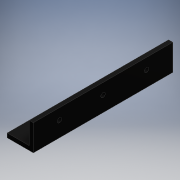
# Autodesk Inventor part: Horn_Bracket
Saved by Autodesk Inventor 2016 (Build 200138000, 138)
## iProperties
Created: 2016-05-21
Part Number: Horn_Bracket
Material: Steel, Cast
Document SubType Name: Modeling
Designer: agmle
Density: 7.85 g/cm^3
Appearance: Glossy - Black
Mass: 1504.55 g
Surface Area: 548.079 cm^2
Volume: 191.662 cm^3
Mounting_Hole_Spacing: 82.800 mm
Mounting_Hole_Diameter: 8.450 mm
Author: agmle
Autodesk Inventor part; units mm, degrees
ref_plane "YZ Plane" through (0, 0, 0) normal (1, 0, 0) x (0, 1, 0)
ref_plane "XZ Plane" through (0, 0, 0) normal (0, 1, 0) x (-1, 0, 0)
ref_plane "XY Plane" through (0, 0, 0) normal (0, 0, 1) x (1, 0, 0)
sketch "Sketch1" plane through (0, 0, 0) normal (0, 1, 0) x (-1, 0, 0)
  line L0 (0, 0) -> (0, 49.7)
  line L1 (0, 49.7) -> (8, 49.7)
  line L2 (8, 49.7) -> (8, 8)
  line L3 (8, 8) -> (49.7, 8)
  line L4 (49.7, 8) -> (49.7, 0)
  line L5 (49.7, 0) -> (0, 0)
  dimension "d0" = 49.7
  dimension "d1" = 8
  constraints: 12 end point, 6 perpendicular, 1 parallel, 1 vertical
  measures "d0" distance between parallel lines of L0 L4
  measures "d1" distance between parallel lines of L0 L2
extrude "Extrusion1" add sketch "Sketch1" along normal blind 265
sketch "Sketch2" plane through (0, 0, 0) normal (0, 0, -1) x (-1, 0, 0)
  line L0 (49.7, 0) -> (0, 0) construction
  line L1 (49.7, 0) -> (49.7, 265) construction
  line L2 (0, 265) -> (49.7, 265) construction
  line L3 (0, 0) -> (0, 265) construction
  line L4 (31, 0) -> (31, 265) construction
  line L5 (0, 265) -> (49.7, 265) construction
  point P0 (31, 231)
  point P1 (31, 205)
  point P2 (31, 60)
  point P3 (31, 34)
  dimension "d4" = 26
  dimension "d5" = 26
  dimension "d6" = 34
  dimension "d7" = 34
  dimension "d8" = 31
  constraints: 6 point on line, 2 end point, 1 perpendicular
  measures "d4" distance of point (31, 34) point (31, 60)
  measures "d5" distance of point (31, 231) point (31, 205)
  measures "d6" distance from line of L2 point (31, 231)
  measures "d7" distance from line of L0 point (31, 34)
  measures "d8" distance between parallel lines of L3 L4
hole "Hole1" at (-31, 231, 0) at (-31, 205, 0) at (-31, 60, 0) at (-31, 34, 0) direction (0, 0, 1) diameter 5.5 depth 8 tip angle 118 clearance for "Hex Head Bolt" size "M5" standard "Ansi Metric M Profile"
sketch "Sketch3" plane through (0, 0, 49.7) normal (1, 0, 0) x (0, 0, -1)
  line L0 (49.7, 0) -> (0, 0) construction
  line L1 (49.7, 0) -> (49.7, 265) construction
  line L2 (0, 265) -> (49.7, 265) construction
  line L3 (0, 0) -> (0, 265) construction
  line L4 (0, 0) -> (41.7, 0) construction
  line L5 (20.8, 0) -> (20.8, 265) construction
  point P0 (20.8, 132.5)
  point P1 (20.8, 215.3)
  point P2 (20.8, 49.7)
  dimension "d16" = 20.8
  dimension "Mounting_Hole_Spacing" = 82.8
  dimension "d18" = 82.8
  constraints: 4 point on line, 2 end point, 1 midpoint, 1 perpendicular
  measures "d16" distance between parallel lines of L3 L5
  measures "Mounting_Hole_Spacing" distance of point (20.8, 132.5) point (20.8, 49.7)
  measures "d18" distance of point (20.8, 215.3) point (20.8, 132.5)
hole "Hole2" at (0, 132.5, 28.9) at (0, 215.3, 28.9) at (0, 49.7, 28.9) direction (-1, 0, 0) diameter 8.45 end through all
equation "\"d4\" = Mount_Hole_Spacing"
equation "\"d5\" = Mount_Hole_Spacing"
equation "\"d7\" = d6"
equation "\"d18\" = Mounting_Hole_Spacing"
equation "\"Mount_Hole_Spacing\" = 26"
body "Solid1"
